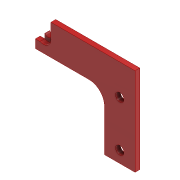
# Autodesk Inventor part: Odometry stop left
Saved by Autodesk Inventor 2020 (Build 240168000, 168)
## iProperties
Created: 2020-03-07
Part Number: Odometry stop left
Material: Generic
Document SubType Name: Modeling
Designer: ball
Density: 1 g/cm^3
Appearance: Default
Author: ball
Autodesk Inventor part; units mm, degrees
ref_plane "YZ Plane" through (0, 0, 0) normal (1, 0, 0) x (0, 1, 0)
ref_plane "XZ Plane" through (0, 0, 0) normal (0, 1, 0) x (-1, 0, 0)
ref_plane "XY Plane" through (0, 0, 0) normal (0, 0, 1) x (1, 0, 0)
ref_plane "Work Plane5" through (0, 0, 0) normal (0, 0, 1) x (1, 0, 0)
sketch "Sketch1" plane through (0, 0, 0) normal (0, 0, 1) x (1, 0, 0)
  arc A0 (-50, 35.3137) -> (-46, 35.3137) centre (-48, 35.3137) ccw construction
  arc A1 (-46, 40) -> (-50, 40) centre (-48, 40) ccw construction
  line L0 (-50, 35.3137) -> (-50, 40) construction
  line L1 (-46, 40) -> (-46, 35.3137) construction
  line L2 (-46.254, 38.8332) -> (-46.254, 35.3137)
  arc A2 (-49.746, 35.3137) -> (-46.254, 35.3137) centre (-48, 35.3137) ccw
  line L3 (-49.746, 35.3137) -> (-49.746, 38.8332)
  arc A3 (-49.746, 38.8332) -> (-46.254, 38.8332) centre (-48, 40) ccw
  point P0 (0, 0)
  dimension "d1" = 4.2
  constraints: 4 end point, 4 point on circle, 2 centre point, 1 coincident
  measures "d1" diameter of A3
extrude "Extrusion1" add sketch "Sketch1" against normal blind 2.5
ref_plane "Work Plane6" through (0, 0, 0) normal (0, 0, 1) x (1, 0, 0)
sketch "Sketch2" plane through (0, 0, 0) normal (0, 0, 1) x (1, 0, 0)
  line L0 (-52.1646, 48) -> (0, 48)
  line L1 (0, 48) -> (0, 2)
  arc A0 (-16, 24) -> (-24, 32) centre (-24, 24) ccw
  circle A1 centre (-8, 8) radius 2.2
  circle A2 centre (-8, 32) radius 2.2
  line L2 (-52.1646, 32) -> (-24, 32)
  line L3 (-16, 24) -> (-16, 2)
  line L4 (0, 2) -> (-16, 2)
  arc A3 (-49.746, 38.8332) -> (-46.254, 38.8332) centre (-48, 40) ccw projected
  line L5 (-52.1646, 48) -> (-52.1646, 32)
  line L6 (-52.1646, 48) -> (-36.1646, 48) construction
  point P0 (-54, 48)
  dimension "d7" = 4.4
  dimension "d8" = 4.4
  dimension "d9" = 24
  dimension "d22" = 48
  dimension "d23" = 90
  dimension "d24" = 46
  dimension "d25" = 16
  dimension "d26" = 8
  dimension "d27" = 8
  constraints: 14 end point, 3 centre point, 3 horizontal, 2 coincident, 2 perpendicular, 2 point on circle, 2 tangent, 1 other
  measures "d7" diameter of A1
  measures "d8" diameter of A2
  measures "d9" distance of A2.centre point (-8, 8)
  measures "d22" distance from line of A3.centre L1
  measures "d23" angle of L5 L6
  measures "d24" distance between parallel lines of L0 L4
  measures "d25" distance from line of L0 A2.centre
  measures "d26" distance from line of L0 A3.centre
  measures "d27" distance from line of L1 A2.centre
extrude "Extrusion2" add sketch "Sketch2" along normal blind 2.5
sketch "Sketch6" plane through (0, 0, 0) normal (0, 0, -1) x (-1, 0, 0)
  arc A0 (46.254, 38.8332) -> (49.746, 38.8332) centre (48, 40) ccw projected
  arc A1 (44, 40) -> (49.746, 36.4012) centre (48, 40) ccw
  line L0 (52.1646, 48) -> (52.1646, 32) projected
  line L1 (49.746, 35.3137) -> (49.746, 38.8332) projected
  line L2 (49.746, 36.4012) -> (52.1646, 36.4012)
  line L3 (52.1646, 36.4012) -> (52.1646, 44)
  line L4 (44, 40) -> (44, 48)
  line L5 (0, 48) -> (52.1646, 48) projected
  line L6 (44, 48) -> (52.1646, 48)
  line L7 (52.1646, 44) -> (52.1646, 48)
  point P0 (0, 0)
  dimension "d31" = 8
  constraints: 10 end point, 4 point on line, 2 collinear, 2 perpendicular, 2 point on circle, 1 centre point, 1 coincident, 1 vertical
  measures "d31" diameter of A1
extrude "Extrusion6" cut sketch "Sketch6" against normal up to surface (2.5 mm away)
body "Solid1"
